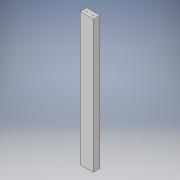
# Autodesk Inventor part: stand_vert
Saved by Autodesk Inventor 2019 (Build 230136000, 136)
## iProperties
Created: 2019-12-27
Part Number: stand_vert
Material: Типовые
Document SubType Name: Modeling
Designer: stepa
Density: 1 g/cm^3
Appearance: По умолчанию
Author: stepa
Autodesk Inventor part; units mm, degrees
ref_plane "YZ Plane" through (0, 0, 0) normal (1, 0, 0) x (0, 1, 0)
ref_plane "XZ Plane" through (0, 0, 0) normal (0, 1, 0) x (-1, 0, 0)
ref_plane "XY Plane" through (0, 0, 0) normal (0, 0, 1) x (1, 0, 0)
sketch "Эскиз1" plane through (0, 0, 0) normal (0, 1, 0) x (-1, 0, 0)
  line L0 (0, 0) -> (-60, 0)
  line L1 (-60, 0) -> (-60, -30)
  line L2 (-60, -30) -> (0, -30)
  line L3 (0, -30) -> (0, 0)
  dimension "d0" = 60
  dimension "d1" = 30
  constraints: 8 end point, 2 parallel, 1 horizontal, 1 perpendicular
  measures "d0" distance of L2.end L1.end
  measures "d1" distance of L1.end L0.end
extrude "Выдавливание1" add sketch "Эскиз1" along normal blind 600
sketch "Эскиз2" plane through (0, 600, 0) normal (0, 1, 0) x (1, 0, 0)
  line L0 (0, 30) -> (0, 0) projected
  point P0 (15, 15)
  point P1 (45, 15)
  point P2 (0, 15)
  dimension "d4" = 30
  dimension "d5" = 15
  constraints: 2 horizontal alignment, 1 midpoint
  measures "d4" distance of point (45, 15) point (15, 15)
  measures "d5" distance from line of L0 point (15, 15)
hole "Отверстие1" at (15, 600, -15) at (45, 600, -15) direction (0, -1, 0) diameter 3 end through all
